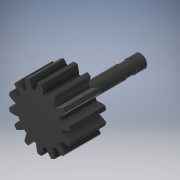
# Autodesk Inventor part: AC06
Saved by Autodesk Inventor 2017 (Build 210142000, 142)
## iProperties
Created: 2019-09-22
Part Number: AC06
Material: ABS Plastic
Document SubType Name: Modeling
Designer: Zach
Density: 1.06 g/cm^3
Appearance: Smooth - Black
Author: Zach
Autodesk Inventor part; units mm, degrees
ref_plane "YZ Plane" through (0, 0, 0) normal (1, 0, 0) x (0, 1, 0)
ref_plane "XZ Plane" through (0, 0, 0) normal (0, 1, 0) x (-1, 0, 0)
ref_plane "XY Plane" through (0, 0, 0) normal (0, 0, 1) x (1, 0, 0)
sketch "Sketch1" plane through (0, 0, 0) normal (0, 0, 1) x (1, 0, 0)
  arc A0 (5.9892, 8.4411) -> (6.9584, 12.5904) centre (-5.202, 13.243) ccw
  arc A1 (6.9584, 12.5904) -> (5.505, 13.2903) centre (0, 0) ccw
  arc A2 (5.505, 13.2903) -> (2.8652, 9.9455) centre (13.5971, 4.1898) ccw
  arc A3 (2.8652, 9.9455) -> (1.7337, 10.2038) centre (0, 0) ccw
  arc A4 (1.7337, 10.2038) -> (0.8066, 14.3627) centre (-10.4327, 9.6744) ccw
  arc A5 (0.8066, 14.3627) -> (-0.8066, 14.3627) centre (0, 0) ccw
  arc A6 (-0.8066, 14.3627) -> (-1.7337, 10.2038) centre (10.4327, 9.6744) ccw
  arc A7 (-1.7337, 10.2038) -> (-2.8652, 9.9455) centre (0, 0) ccw
  arc A8 (-2.8652, 9.9455) -> (-5.505, 13.2903) centre (-13.5971, 4.1898) ccw
  arc A9 (-5.505, 13.2903) -> (-6.9584, 12.5904) centre (0, 0) ccw
  arc A10 (-6.9584, 12.5904) -> (-5.9892, 8.4411) centre (5.202, 13.243) ccw
  arc A11 (-5.9892, 8.4411) -> (-6.8967, 7.7174) centre (0, 0) ccw
  arc A12 (-6.8967, 7.7174) -> (-10.7263, 9.5856) centre (-14.0685, -2.1247) ccw
  arc A13 (-10.7263, 9.5856) -> (-11.7321, 8.3244) centre (0, 0) ccw
  arc A14 (-11.7321, 8.3244) -> (-9.0586, 5.0065) centre (-1.0591, 14.1885) ccw
  arc A15 (-9.0586, 5.0065) -> (-9.5622, 3.9608) centre (0, 0) ccw
  arc A16 (-9.5622, 3.9608) -> (-13.8231, 3.9824) centre (-11.7534, -8.0184) ccw
  arc A17 (-13.8231, 3.9824) -> (-14.1821, 2.4096) centre (0, 0) ccw
  arc A18 (-14.1821, 2.4096) -> (-10.3337, 0.5803) centre (-7.1104, 12.3239) ccw
  arc A19 (-10.3337, 0.5803) -> (-10.3337, -0.5803) centre (0, 0) ccw
  arc A20 (-10.3337, -0.5803) -> (-14.1821, -2.4096) centre (-7.1104, -12.3239) ccw
  arc A21 (-14.1821, -2.4096) -> (-13.8231, -3.9824) centre (0, 0) ccw
  arc A22 (-13.8231, -3.9824) -> (-9.5622, -3.9608) centre (-11.7534, 8.0184) ccw
  arc A23 (-9.5622, -3.9608) -> (-9.0586, -5.0065) centre (0, 0) ccw
  arc A24 (-9.0586, -5.0065) -> (-11.7321, -8.3244) centre (-1.0591, -14.1885) ccw
  arc A25 (-11.7321, -8.3244) -> (-10.7263, -9.5856) centre (0, 0) ccw
  arc A26 (-10.7263, -9.5856) -> (-6.8967, -7.7174) centre (-14.0685, 2.1247) ccw
  arc A27 (-6.8967, -7.7174) -> (-5.9892, -8.4411) centre (0, 0) ccw
  arc A28 (-5.9892, -8.4411) -> (-6.9584, -12.5904) centre (5.202, -13.243) ccw
  arc A29 (-6.9584, -12.5904) -> (-5.505, -13.2903) centre (0, 0) ccw
  arc A30 (-5.505, -13.2903) -> (-2.8652, -9.9455) centre (-13.5971, -4.1898) ccw
  arc A31 (-2.8652, -9.9455) -> (-1.7337, -10.2038) centre (0, 0) ccw
  arc A32 (-1.7337, -10.2038) -> (-0.8066, -14.3627) centre (10.4327, -9.6744) ccw
  arc A33 (-0.8066, -14.3627) -> (0.8066, -14.3627) centre (0, 0) ccw
  arc A34 (0.8066, -14.3627) -> (1.7337, -10.2038) centre (-10.4327, -9.6744) ccw
  arc A35 (1.7337, -10.2038) -> (2.8652, -9.9455) centre (0, 0) ccw
  arc A36 (2.8652, -9.9455) -> (5.505, -13.2903) centre (13.5971, -4.1898) ccw
  arc A37 (5.505, -13.2903) -> (6.9584, -12.5904) centre (0, 0) ccw
  arc A38 (6.9584, -12.5904) -> (5.9892, -8.4411) centre (-5.202, -13.243) ccw
  arc A39 (5.9892, -8.4411) -> (6.8967, -7.7174) centre (0, 0) ccw
  arc A40 (6.8967, -7.7174) -> (10.7263, -9.5856) centre (14.0685, 2.1247) ccw
  arc A41 (10.7263, -9.5856) -> (11.7321, -8.3244) centre (0, 0) ccw
  arc A42 (11.7321, -8.3244) -> (9.0586, -5.0065) centre (1.0591, -14.1885) ccw
  arc A43 (9.0586, -5.0065) -> (9.5622, -3.9608) centre (0, 0) ccw
  arc A44 (9.5622, -3.9608) -> (13.8231, -3.9824) centre (11.7534, 8.0184) ccw
  arc A45 (13.8231, -3.9824) -> (14.1821, -2.4096) centre (0, 0) ccw
  arc A46 (14.1821, -2.4096) -> (10.3337, -0.5803) centre (7.1104, -12.3239) ccw
  arc A47 (10.3337, -0.5803) -> (10.3337, 0.5803) centre (0, 0) ccw
  arc A48 (10.3337, 0.5803) -> (14.1821, 2.4096) centre (7.1104, 12.3239) ccw
  arc A49 (14.1821, 2.4096) -> (13.8231, 3.9824) centre (0, 0) ccw
  arc A50 (13.8231, 3.9824) -> (9.5622, 3.9608) centre (11.7534, -8.0184) ccw
  arc A51 (9.5622, 3.9608) -> (9.0586, 5.0065) centre (0, 0) ccw
  arc A52 (9.0586, 5.0065) -> (11.7321, 8.3244) centre (1.0591, 14.1885) ccw
  arc A53 (11.7321, 8.3244) -> (10.7263, 9.5856) centre (0, 0) ccw
  arc A54 (10.7263, 9.5856) -> (6.8967, 7.7174) centre (14.0685, -2.1247) ccw
  arc A55 (6.8967, 7.7174) -> (5.9892, 8.4411) centre (0, 0) ccw
  constraints: 112 point on circle, 56 centre point
extrude "Extrusion1" add sketch "Sketch1" along normal blind 16
sketch "Sketch2" plane through (0, 0, 0) normal (0, 0, -1) x (-1, 0, 0)
  circle A0 centre (0, 0) radius 2.925
  dimension "d2" = 5.85
  constraints: 1 centre point, 1 coincident
  measures "d2" diameter of A0
extrude "Extrusion2" add sketch "Sketch2" along normal blind 20
sketch "Sketch4" plane through (0, 0, -20) normal (0, 0, -1) x (-1, 0, 0)
  circle A0 centre (0, 0) radius 2.675
  dimension "d8" = 5.35
  constraints: 1 centre point, 1 coincident
  measures "d8" diameter of A0
extrude "Extrusion4" add sketch "Sketch4" along normal blind 4.5
sketch "Sketch7" plane through (0, 0, -24.5) normal (0, 0, -1) x (-1, 0, 0)
  circle A0 centre (0, 0) radius 2.925 projected
extrude "Extrusion6" add sketch "Sketch7" along normal blind 4.5
sketch "Sketch11" plane through (0, 0, 16) normal (0, 0, 1) x (1, 0, 0)
  circle A0 centre (0, 0) radius 14
  circle A1 centre (0, 0) radius 25
  dimension "d23" = 28
  dimension "d24" = 50
  constraints: 2 centre point, 2 coincident
  measures "d23" diameter of A0
  measures "d24" diameter of A1
extrude "Extrusion9" cut sketch "Sketch11" against normal through all
sketch "Sketch12" plane through (0, 0, 16) normal (0, 0, 1) x (1, 0, 0)
  arc A0 (13.8311, 2.1684) -> (13.4022, 4.0474) centre (0, 0) ccw projected
  arc A1 (13.4022, 4.0474) -> (9.5622, 3.9608) centre (11.7534, -8.0184) ccw projected
  arc A2 (9.5622, 3.9608) -> (9.0586, 5.0065) centre (0, 0) ccw projected
  arc A3 (9.0586, 5.0065) -> (11.5205, 7.9547) centre (1.0591, 14.1885) ccw projected
  arc A4 (11.5205, 7.9547) -> (10.3188, 9.4616) centre (0, 0) ccw projected
  arc A5 (10.3188, 9.4616) -> (6.8967, 7.7174) centre (14.0685, -2.1247) ccw projected
  arc A6 (6.8967, 7.7174) -> (5.9892, 8.4411) centre (0, 0) ccw projected
  arc A7 (5.9892, 8.4411) -> (6.9282, 12.1655) centre (-5.202, 13.243) ccw projected
  arc A8 (6.9282, 12.1655) -> (5.1917, 13.0018) centre (0, 0) ccw projected
  arc A9 (5.1917, 13.0018) -> (2.8652, 9.9455) centre (13.5971, 4.1898) ccw projected
  arc A10 (2.8652, 9.9455) -> (1.7337, 10.2038) centre (0, 0) ccw projected
  arc A11 (1.7337, 10.2038) -> (0.9637, 13.9668) centre (-10.4327, 9.6744) ccw projected
  arc A12 (0.9637, 13.9668) -> (-0.9637, 13.9668) centre (0, 0) ccw projected
  arc A13 (-0.9637, 13.9668) -> (-1.7337, 10.2038) centre (10.4327, 9.6744) ccw projected
  arc A14 (-1.7337, 10.2038) -> (-2.8652, 9.9455) centre (0, 0) ccw projected
  arc A15 (-2.8652, 9.9455) -> (-5.1917, 13.0018) centre (-13.5971, 4.1898) ccw projected
  arc A16 (-5.1917, 13.0018) -> (-6.9282, 12.1655) centre (0, 0) ccw projected
  arc A17 (-6.9282, 12.1655) -> (-5.9892, 8.4411) centre (5.202, 13.243) ccw projected
  arc A18 (-5.9892, 8.4411) -> (-6.8967, 7.7174) centre (0, 0) ccw projected
  arc A19 (-6.8967, 7.7174) -> (-10.3188, 9.4616) centre (-14.0685, -2.1247) ccw projected
  arc A20 (-10.3188, 9.4616) -> (-11.5205, 7.9547) centre (0, 0) ccw projected
  arc A21 (-11.5205, 7.9547) -> (-9.0586, 5.0065) centre (-1.0591, 14.1885) ccw projected
  arc A22 (-9.0586, 5.0065) -> (-9.5622, 3.9608) centre (0, 0) ccw projected
  arc A23 (-9.5622, 3.9608) -> (-13.4022, 4.0474) centre (-11.7534, -8.0184) ccw projected
  arc A24 (-13.4022, 4.0474) -> (-13.8311, 2.1684) centre (0, 0) ccw projected
  arc A25 (-13.8311, 2.1684) -> (-10.3337, 0.5803) centre (-7.1104, 12.3239) ccw projected
  arc A26 (-10.3337, 0.5803) -> (-10.3337, -0.5803) centre (0, 0) ccw projected
  arc A27 (-10.3337, -0.5803) -> (-13.8311, -2.1684) centre (-7.1104, -12.3239) ccw projected
  arc A28 (-13.8311, -2.1684) -> (-13.4022, -4.0474) centre (0, 0) ccw projected
  arc A29 (-13.4022, -4.0474) -> (-9.5622, -3.9608) centre (-11.7534, 8.0184) ccw projected
  arc A30 (-9.5622, -3.9608) -> (-9.0586, -5.0065) centre (0, 0) ccw projected
  arc A31 (-9.0586, -5.0065) -> (-11.5205, -7.9547) centre (-1.0591, -14.1885) ccw projected
  arc A32 (-11.5205, -7.9547) -> (-10.3188, -9.4616) centre (0, 0) ccw projected
  arc A33 (-10.3188, -9.4616) -> (-6.8967, -7.7174) centre (-14.0685, 2.1247) ccw projected
  arc A34 (-6.8967, -7.7174) -> (-5.9892, -8.4411) centre (0, 0) ccw projected
  arc A35 (-5.9892, -8.4411) -> (-6.9282, -12.1655) centre (5.202, -13.243) ccw projected
  arc A36 (-6.9282, -12.1655) -> (-5.1917, -13.0018) centre (0, 0) ccw projected
  arc A37 (-5.1917, -13.0018) -> (-2.8652, -9.9455) centre (-13.5971, -4.1898) ccw projected
  arc A38 (-2.8652, -9.9455) -> (-1.7337, -10.2038) centre (0, 0) ccw projected
  arc A39 (-1.7337, -10.2038) -> (-0.9637, -13.9668) centre (10.4327, -9.6744) ccw projected
  arc A40 (-0.9637, -13.9668) -> (0.9637, -13.9668) centre (0, 0) ccw projected
  arc A41 (0.9637, -13.9668) -> (1.7337, -10.2038) centre (-10.4327, -9.6744) ccw projected
  arc A42 (1.7337, -10.2038) -> (2.8652, -9.9455) centre (0, 0) ccw projected
  arc A43 (2.8652, -9.9455) -> (5.1917, -13.0018) centre (13.5971, -4.1898) ccw projected
  arc A44 (5.1917, -13.0018) -> (6.9282, -12.1655) centre (0, 0) ccw projected
  arc A45 (6.9282, -12.1655) -> (5.9892, -8.4411) centre (-5.202, -13.243) ccw projected
  arc A46 (5.9892, -8.4411) -> (6.8967, -7.7174) centre (0, 0) ccw projected
  arc A47 (6.8967, -7.7174) -> (10.3188, -9.4616) centre (14.0685, 2.1247) ccw projected
  arc A48 (10.3188, -9.4616) -> (11.5205, -7.9547) centre (0, 0) ccw projected
  arc A49 (11.5205, -7.9547) -> (9.0586, -5.0065) centre (1.0591, -14.1885) ccw projected
  arc A50 (9.0586, -5.0065) -> (9.5622, -3.9608) centre (0, 0) ccw projected
  arc A51 (9.5622, -3.9608) -> (13.4022, -4.0474) centre (11.7534, 8.0184) ccw projected
  arc A52 (13.4022, -4.0474) -> (13.8311, -2.1684) centre (0, 0) ccw projected
  arc A53 (13.8311, -2.1684) -> (10.3337, -0.5803) centre (7.1104, -12.3239) ccw projected
  arc A54 (10.3337, -0.5803) -> (10.3337, 0.5803) centre (0, 0) ccw projected
  arc A55 (10.3337, 0.5803) -> (13.8311, 2.1684) centre (7.1104, 12.3239) ccw projected
  arc A56 (6.7169, 12.055) -> (5.2371, 12.7677) centre (0, 0) ccw
  arc A57 (5.7403, 8.3709) -> (6.7169, 12.055) centre (-5.202, 13.243) ccw
  arc A58 (6.8837, 7.4591) -> (5.7403, 8.3709) centre (0, 0) ccw
  arc A59 (10.2581, 9.231) -> (6.8837, 7.4591) centre (14.0685, -2.1247) ccw
  arc A60 (11.2822, 7.9468) -> (10.2581, 9.231) centre (0, 0) ccw
  arc A61 (8.8038, 5.0513) -> (11.2822, 7.9468) centre (1.0591, 14.1885) ccw
  arc A62 (9.4383, 3.7337) -> (8.8038, 5.0513) centre (0, 0) ccw
  arc A63 (13.2474, 3.866) -> (9.4383, 3.7337) centre (11.7534, -8.0184) ccw
  arc A64 (13.6129, 2.2647) -> (13.2474, 3.866) centre (0, 0) ccw
  arc A65 (10.1236, 0.7312) -> (13.6129, 2.2647) centre (7.1104, 12.3239) ccw
  arc A66 (10.1236, -0.7312) -> (10.1236, 0.7312) centre (0, 0) ccw
  arc A67 (13.6129, -2.2647) -> (10.1236, -0.7312) centre (7.1104, -12.3239) ccw
  arc A68 (13.2474, -3.866) -> (13.6129, -2.2647) centre (0, 0) ccw
  arc A69 (9.4383, -3.7337) -> (13.2474, -3.866) centre (11.7534, 8.0184) ccw
  arc A70 (8.8038, -5.0513) -> (9.4383, -3.7337) centre (0, 0) ccw
  arc A71 (11.2822, -7.9468) -> (8.8038, -5.0513) centre (1.0591, -14.1885) ccw
  arc A72 (10.2581, -9.231) -> (11.2822, -7.9468) centre (0, 0) ccw
  arc A73 (6.8837, -7.4591) -> (10.2581, -9.231) centre (14.0685, 2.1247) ccw
  arc A74 (5.7403, -8.3709) -> (6.8837, -7.4591) centre (0, 0) ccw
  arc A75 (6.7169, -12.055) -> (5.7403, -8.3709) centre (-5.202, -13.243) ccw
  arc A76 (5.2371, -12.7677) -> (6.7169, -12.055) centre (0, 0) ccw
  arc A77 (2.9656, -9.7071) -> (5.2371, -12.7677) centre (13.5971, -4.1898) ccw
  arc A78 (1.5398, -10.0325) -> (2.9656, -9.7071) centre (0, 0) ccw
  arc A79 (0.8212, -13.7755) -> (1.5398, -10.0325) centre (-10.4327, -9.6744) ccw
  arc A80 (-0.8212, -13.7755) -> (0.8212, -13.7755) centre (0, 0) ccw
  arc A81 (-1.5398, -10.0325) -> (-0.8212, -13.7755) centre (10.4327, -9.6744) ccw
  arc A82 (-2.9656, -9.7071) -> (-1.5398, -10.0325) centre (0, 0) ccw
  arc A83 (-5.2371, -12.7677) -> (-2.9656, -9.7071) centre (-13.5971, -4.1898) ccw
  arc A84 (-6.7169, -12.055) -> (-5.2371, -12.7677) centre (0, 0) ccw
  arc A85 (-5.7403, -8.3709) -> (-6.7169, -12.055) centre (5.202, -13.243) ccw
  arc A86 (-6.8837, -7.4591) -> (-5.7403, -8.3709) centre (0, 0) ccw
  arc A87 (-10.2581, -9.231) -> (-6.8837, -7.4591) centre (-14.0685, 2.1247) ccw
  arc A88 (-11.2822, -7.9468) -> (-10.2581, -9.231) centre (0, 0) ccw
  arc A89 (-8.8038, -5.0513) -> (-11.2822, -7.9468) centre (-1.0591, -14.1885) ccw
  arc A90 (-9.4383, -3.7337) -> (-8.8038, -5.0513) centre (0, 0) ccw
  arc A91 (-13.2474, -3.866) -> (-9.4383, -3.7337) centre (-11.7534, 8.0184) ccw
  arc A92 (-13.6129, -2.2647) -> (-13.2474, -3.866) centre (0, 0) ccw
  arc A93 (-10.1236, -0.7312) -> (-13.6129, -2.2647) centre (-7.1104, -12.3239) ccw
  arc A94 (-10.1236, 0.7312) -> (-10.1236, -0.7312) centre (0, 0) ccw
  arc A95 (-13.6129, 2.2647) -> (-10.1236, 0.7312) centre (-7.1104, 12.3239) ccw
  arc A96 (-13.2474, 3.866) -> (-13.6129, 2.2647) centre (0, 0) ccw
  arc A97 (-9.4383, 3.7337) -> (-13.2474, 3.866) centre (-11.7534, -8.0184) ccw
  arc A98 (-8.8038, 5.0513) -> (-9.4383, 3.7337) centre (0, 0) ccw
  arc A99 (-11.2822, 7.9468) -> (-8.8038, 5.0513) centre (-1.0591, 14.1885) ccw
  arc A100 (-10.2581, 9.231) -> (-11.2822, 7.9468) centre (0, 0) ccw
  arc A101 (-6.8837, 7.4591) -> (-10.2581, 9.231) centre (-14.0685, -2.1247) ccw
  arc A102 (-5.7403, 8.3709) -> (-6.8837, 7.4591) centre (0, 0) ccw
  arc A103 (-6.7169, 12.055) -> (-5.7403, 8.3709) centre (5.202, 13.243) ccw
  arc A104 (-5.2371, 12.7677) -> (-6.7169, 12.055) centre (0, 0) ccw
  arc A105 (-2.9656, 9.7071) -> (-5.2371, 12.7677) centre (-13.5971, 4.1898) ccw
  arc A106 (-1.5398, 10.0325) -> (-2.9656, 9.7071) centre (0, 0) ccw
  arc A107 (-0.8212, 13.7755) -> (-1.5398, 10.0325) centre (10.4327, 9.6744) ccw
  arc A108 (0.8212, 13.7755) -> (-0.8212, 13.7755) centre (0, 0) ccw
  arc A109 (1.5398, 10.0325) -> (0.8212, 13.7755) centre (-10.4327, 9.6744) ccw
  arc A110 (2.9656, 9.7071) -> (1.5398, 10.0325) centre (0, 0) ccw
  arc A111 (5.2371, 12.7677) -> (2.9656, 9.7071) centre (13.5971, 4.1898) ccw
  dimension "d27" = 0.2
  constraints: 112 point on circle, 56 centre point, 55 other
  measures "d27" radial gap between concentric circles of A8 A56
extrude "Extrusion10" cut sketch "Sketch12" against normal through all
body "Solid1"
